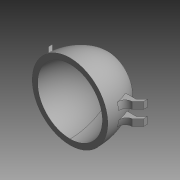
# Autodesk Inventor part: top-round
Saved by Autodesk Inventor 2014 SP2 (Build 180246200, 246)
## iProperties
Created: 2014-11-27
Part Number: top-round
Material: Generic
Document SubType Name: Modeling
Designer: No
Density: 1 g/cm^3
Appearance: Default
Mass: 21.7765 g
Surface Area: 119.721 cm^2
Volume: 21.7765 cm^3
Author: No
Autodesk Inventor part; units mm, degrees
ref_plane "XZ Plane" through (0, 0, 0) normal (0, 1, 0) x (-1, 0, 0)
ref_plane "XY Plane" through (0, 0, 0) normal (0, 0, 1) x (1, 0, 0)
sketch "Sketch1" plane through (0, 0, 0) normal (1, 0, 0) x (0, 1, 0)
  ellipse E0 centre (0, 0) end of major axis (-37, 0) minor radius 28 (0, -28) -> (37, 0) ccw
  line L0 (37, 0) -> (0, 0)
  line L1 (0, 0) -> (0, -28)
  dimension "outer_semimajor_axis" = 37
  dimension "outer_semiminor_axis" = 28
  constraints: 4 end point, 1 coincident, 1 horizontal, 1 vertical, 4 other
revolve "Revolution1" add sketch "Sketch1" angle 360 about axis through (0, 37, 0) along (0, -1, 0)
ref_plane "Work Plane1" through (19.6, 0, 0) normal (1, 0, 0) x (0, 1, 0)
sketch "Sketch5" plane through (19.6, 0, 0) normal (1, 0, 0) x (0, 1, 0)
  ellipse E0 centre (0, 0) end of major axis (37, 0) minor radius 28 (0, -28) -> (37, 0) ccw projected
  line L0 (0, 28) -> (0, -28) projected
  line L1 (18, 8) -> (15, 8)
  line L2 (15, 8) -> (15, 3)
  line L3 (15, 3) -> (18, 3)
  line L4 (18, 3) -> (18, 8)
  line L5 (0, -19.996) -> (0, 19.996) projected
  dimension "hook_height" = 3
  dimension "hook_width" = 5
  dimension "hook_from_bottom" = 15
  dimension "hook_from_center" = 3
  constraints: 8 end point, 2 parallel, 1 horizontal, 1 perpendicular, 1 vertical alignment, 1 other
  measures "hook_height" distance of L3.end L2.end
  measures "hook_width" distance of L2.end L1.end
  measures "hook_from_bottom" distance between parallel lines of L0 L2
  measures "hook_from_center" distance from line of point (0, 0) L3
extrude "Extrusion3" add sketch "Sketch5" along normal blind 11.4
sketch "Sketch6" plane through (23.1182, 18, 8) normal (0, 0, 1) x (1, 0, 0)
  line L0 (7.8818, 0) -> (7.8818, -3) projected
  line L1 (0, 0) -> (7.8818, 0) projected
  line L2 (7.8818, 0) -> (12.1244, 4.2426)
  line L3 (7.8818, 0) -> (13.8818, 0) construction
  line L4 (12.1244, 4.2426) -> (12.1244, 1.2426)
  line L5 (12.1244, 1.2426) -> (7.8818, -3)
  point P0 (-23.1182, -18)
  dimension "d24" = 6
  dimension "d25" = 45
  dimension "d26" = 3
  constraints: 8 end point, 1 equal length, 1 horizontal, 1 perpendicular
  measures "d24" distance of L0.start L2.end
  measures "d25" angle of L3 L2
  measures "d26" distance of L2.end L4.end
extrude "Extrusion4" add sketch "Sketch6" against normal up to surface (5 mm away)
fillet "Fillet1" radius 5 1 edges at (24.9918, 15, 5.5277)
mirror "Mirror5" about plane through (0, 0, 0) normal (0, 0, 1) of "Extrusion3", "Extrusion4", "Fillet1"
mirror "Mirror6" about plane through (0, 0, 0) normal (1, 0, 0) of "Extrusion3", "Extrusion4", "Fillet1", "Mirror5"
sketch "Sketch2" plane through (0, 0, 0) normal (1, 0, 0) x (0, 1, 0)
  ellipse E0 centre (0, 0) end of major axis (33, 0) minor radius 24 (0, -24) -> (33, 0) ccw
  line L0 (0, 0) -> (33, 0)
  line L1 (0, 0) -> (0, -24)
  dimension "inner_semimajor_axis" = 33
  dimension "inner_semiminor_axis" = 24
  constraints: 4 end point, 1 coincident, 1 horizontal, 1 perpendicular, 4 other
revolve "Revolution2" cut sketch "Sketch2" angle 360 about axis through (0, 0, 0) along (0, 1, 0)
ref_plane "Work Plane3" through (0, 29.6, 0) normal (0, -1, 0) x (1, 0, 0)
sketch "Sketch12" plane through (0, 0, 0) normal (1, 0, 0) x (0, 1, 0)
  line L0 (0, -28) -> (0, -24) projected
  line L1 (0, 24) -> (0, 28) projected
  line L2 (29.6, -49.7645) -> (29.6, 49.7645) projected
  line L3 (37, 0) -> (29.6, 0)
  line L4 (29.6, 0) -> (29.6, -28)
  line L5 (29.6, -28) -> (37, -28)
  line L6 (37, -28) -> (37, 0)
  line L7 (-9.7567, 0) -> (51.9956, 0) projected
  point P0 (0, 0)
  dimension "d45" = 7.4
  dimension "d46" = 28
  constraints: 8 end point, 2 parallel, 1 horizontal, 1 perpendicular, 1 point on line, 4 other
  measures "d45" distance of L3.start L3.end
  measures "d46" distance of L5.end L3.start
revolve "Revolution3" cut sketch "Sketch12" angle 360 about axis through (0, 0, 0) along (0, 1, 0)
fillet "Fillet2" radius 5 1 edges at (-0.0005, 29.6, 16.8)
equation "\"d26\" = hook_height"
equation "\"d27\" = 0.3 * outer_semiminor_axis"
equation "\"d45\" = outer_semimajor_axis + cut_plane_start"
equation "\"d46\" = outer_semiminor_axis"
equation "\"hook_start_plane_from_center\" = 0.7 * outer_semiminor_axis"
equation "\"cut_plane_start\" = -0.8 * outer_semimajor_axis"
body "Solid1"
